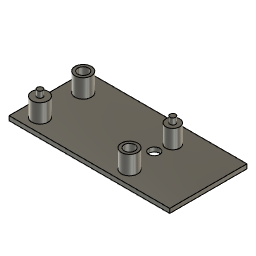
Base placa TTGO LoRa32 v1 (Autodesk Fusion 360 design; units mm, degrees)
Autodesk Fusion 360 part; units mm, degrees
sketch "Boceto1" plane through (0, 0, 0) normal (0, 0, 1) x (1, 0, 0)
  line L0 (0, 0) -> (52, 0)
  line L1 (52, 0) -> (52, 25)
  line L2 (52, 25) -> (0, 25)
  line L3 (0, 25) -> (0, 0)
  line L4 (0, 25) -> (0, 20.5) construction
  line L5 (0, 25) -> (5.5, 25) construction
  line L6 (0, 20.5) -> (8, 20.5) construction
  line L7 (5.5, 25) -> (5.5, 19) construction
  circle A0 centre (5.5, 20.5) radius 1.75
  circle A1 centre (5.5, 20.5) radius 2.65
  line L8 (5.5, 25) -> (20, 25) construction
  line L9 (20, 25) -> (20, 0) construction
  circle A2 centre (34.5, 20.5) radius 2.65
  circle A3 centre (34.5, 20.5) radius 1.75
  line L10 (0, 20.5) -> (0, 13.5) construction
  line L11 (0, 13.5) -> (20.7832, 13.5) construction
  circle A4 centre (5.5, 6.5) radius 2.65
  circle A5 centre (5.5, 6.5) radius 1.75
  circle A6 centre (34.5, 6.5) radius 1.75
  circle A7 centre (34.5, 6.5) radius 2.25
  dimension "d5" = 52
  dimension "d6" = 25
  dimension "d9" = 4.5
  dimension "d10" = 5.5
  dimension "d17" = 3.5
  dimension "d18" = 5.3
  dimension "d19" = 14.5
  dimension "d20" = 7
  dimension "d38" = 4.5
  constraint horizontal L0
  constraint vertical L1
  constraint horizontal L2
  constraint vertical L3
  constraint coincident L0.start L3.end
  constraint perpendicular L2 L4
  constraint perpendicular L4 L5
  constraint perpendicular L4 L6
  constraint perpendicular L6 L7
  constraint coincident L6 A0.centre
  constraint coincident L7 A0.centre
  constraint concentric A0 A1
  constraint perpendicular L7 L8
  constraint coincident L0 L9.end
  constraint perpendicular L0 L9
  constraint symmetric A0 L9 A3
  constraint symmetric A1 L9 A2
  constraint perpendicular L9 L11
  constraint symmetric A0 L11 A5
  constraint symmetric A1 L11 A4
  constraint symmetric L9 A5 A6
  constraint concentric A6 A7
  measures "d5" distance of L0.start L0.end
  measures "d6" distance of L0.start L2.end
  measures "d9" distance of L2.end L4.end
  measures "d10" distance of L2.end L5.end
  measures "d17" diameter of A0
  measures "d18" diameter of A1
  measures "d19" distance of L5.end L8.end
  measures "d20" distance of L4.end L10.end
  measures "d38" diameter of A7
extrude "Extruir1" add sketch "Boceto1" against normal blind 1.4 contours L0 L1 L2 L3 | A6 | A7
extrude "Extruir2" add sketch "Boceto1" against normal blind 7.4 contours A0 | A1 | A2 | A4 | A6 | A7
move_body "Desplazar1" bodies 1 to x (1, 0, 0) y (0, -1, 0) z (0, 0, -1) at (0, 25, 0)
sketch "Boceto2" plane through (0, 0, 1.4) normal (0, 0, 1) x (-1, 0, 0)
  circle A0 centre (-5.5, -18.5) radius 2.65
  circle A1 centre (-34.5, -4.5) radius 2.65
  circle A2 centre (-5.5, -4.5) radius 2.65
  line L0 (0, -25) -> (0, 0)
  line L1 (0, 0) -> (-52, 0)
  line L2 (-52, 0) -> (-52, -25)
  line L3 (-52, -25) -> (0, -25)
  line L4 (0, -25) -> (-33.5, -25) construction
  line L5 (-33.5, -25) -> (-33.5, -13.5) construction
  line L6 (-33.5, -13.5) -> (0, -13.5) construction
  line L7 (0, -13.5) -> (0, -25) construction
  circle A3 centre (-33.5, -13.5) radius 1.75
  circle A4 centre (-34.5, -18.5) radius 2.25
  dimension "d27" = 33.5
  dimension "d28" = 11.5
  dimension "d30" = 3.5
  constraint horizontal L4
  constraint vertical L5
  constraint horizontal L6
  constraint vertical L7
  constraint coincident L0.start L3.end
  constraint coincident L5.end L6.start
  measures "d27" distance of L0.start L4.end
  measures "d28" distance of L0.start L6.end
  measures "d30" diameter of A3
extrude "Extruir3" cut sketch "Boceto2" against normal blind 1.4 contours A3
ref_plane "PlanoDeObra1" through (34.5, 18.5, 7.4) normal (0, 0, 1) x (-1, 0, 0)
sketch "Boceto3" plane through (34.5, 18.5, 7.4) normal (0, 0, 1) x (1, 0, 0)
  circle A0 centre (0, 0) radius 0.9
  circle A1 centre (-29, -14) radius 0.9
  dimension "d34" = 1.8
  dimension "d35" = 1.8
  constraint coincident A0.centre origin
  measures "d34" diameter of A0
  measures "d35" diameter of A1
extrude "Extruir4" add sketch "Boceto3" along normal blind 2
equation "largoPlaca = 52 mm"
equation "anchoPlaca = 25 mm"
equation "distanciaTornillosLargo = 29 mm"
equation "distanciaTornillosAncho = 14 mm"
equation "d5 = largoPlaca"
equation "d6 = anchoPlaca"
equation "distanciaAgujeroLargo = 5.5 mm"
equation "distanciaAgujeroCorto = 4.5 mm"
equation "d9 = distanciaAgujeroCorto"
equation "d10 = distanciaAgujeroLargo"
equation "diametroTornillo = 2 mm"
equation "diametroInserto = 3.5 mm"
equation "largoInserto = 6 mm"
equation "grosorPlaca = 1.4 mm"
equation "grosorColumna = 0.9 mm"
equation "d17 = diametroInserto"
equation "d18 = diametroInserto + grosorColumna * 2"
equation "d19 = distanciaTornillosLargo / 2"
equation "d20 = distanciaTornillosAncho / 2"
equation "d21 = -grosorPlaca"
equation "d23 = -grosorPlaca - largoInserto"
equation "distanciaTornilloAncho = 33.5 mm"
equation "distanciaTornilloLargo = 11.5 mm"
equation "d27 = distanciaTornilloAncho"
equation "d28 = distanciaTornilloLargo"
equation "diametroTornilloCaja = 3.5 mm"
equation "d30 = diametroTornilloCaja"
equation "d31 = -grosorPlaca"
equation "d34 = diametroTornillo - 0.2 mm"
equation "d35 = diametroTornillo - 0.2 mm"
named bodies: "Base Placa TTGO LoRa"
